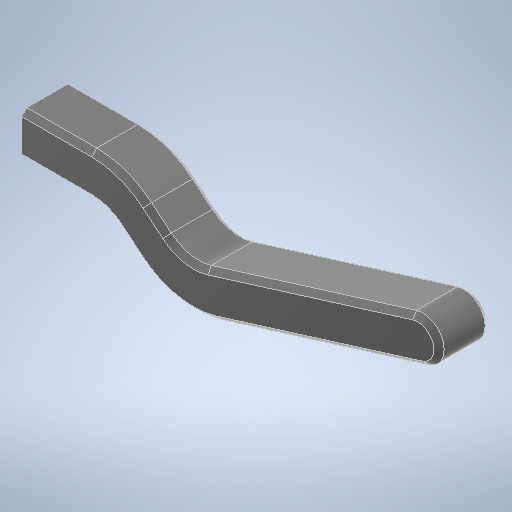
# Autodesk Inventor part: Robot_support
Saved by Autodesk Inventor 2025.2 (Build 292293000, 293)
## iProperties
Created: 2025-02-28
Part Number: Robot_support
Material: Generic
Document SubType Name: Modeling
Designer: Sergio Quintero
Density: 1 g/cm^3
Appearance: Smooth - Black
Author: Sergio Quintero
Autodesk Inventor part; units mm, degrees
ref_plane "YZ Plane" through (0, 0, 0) normal (1, 0, 0) x (0, 1, 0)
ref_plane "XZ Plane" through (0, 0, 0) normal (0, 1, 0) x (-1, 0, 0)
ref_plane "XY Plane" through (0, 0, 0) normal (0, 0, 1) x (1, 0, 0)
sketch "Sketch1" plane through (0, 0, 0) normal (0, 0, 1) x (1, 0, 0)
  line L0 (25, -12.5) -> (-25, -12.5)
  line L1 (-25, -12.5) -> (-25, 12.5)
  line L2 (-25, 12.5) -> (25, 12.5)
  line L3 (25, -12.5) -> (-25, 12.5) construction
  line L4 (-25, -12.5) -> (25, 12.5) construction
  line L5 (25, 12.5) -> (70, 12.5) construction
  line L6 (70, 12.5) -> (70, -17.5) construction
  line L7 (70, -17.5) -> (70, 27.5) construction
  line L8 (70, 27.5) -> (215, 27.5) construction
  line L9 (25, -12.5) -> (64.4199, -45.408)
  line L10 (70, -17.5) -> (41.0213, 6.6916)
  line L11 (70, -17.5) -> (215, 27.5)
  line L12 (215, 27.5) -> (222.41, 3.6234)
  line L13 (222.41, 3.6234) -> (77.41, -41.3766)
  line L14 (41.0213, 6.6916) -> (34.0635, 12.5)
  line L15 (25, 12.5) -> (34.0635, 12.5)
  line L16 (77.41, -41.3766) -> (64.4199, -45.408)
  point P0 (0, 0)
  dimension "d3" = 30
  dimension "d5" = 50
  dimension "d6" = 25
  dimension "d7" = 45
  dimension "d8" = 45
  dimension "d9" = 145
  dimension "d12" = 25
  dimension "d13" = 25
  constraints: 34 end point, 4 perpendicular, 3 parallel, 2 collinear, 2 horizontal, 2 midpoint, 1 point on line, 1 vertical
  measures "d3" distance of L6.end L5.end
  measures "d5" distance from line of L2.end L1
  measures "d6" distance between parallel lines of L0 L2
  measures "d7" distance from line of L6 L2.end
  measures "d8" distance of L6.end L7.end
  measures "d9" distance of L7.end L8.end
  measures "d12" distance of L8.end L12.end
  measures "d13" distance between parallel lines of L9 L10
extrude "Extrusion1" add sketch "Sketch1" along normal mid plane 30
fillet "Fillet1" radius 50 1 edges at (34.0635, 12.5, 0)
fillet "Fillet2" radius 25 1 edges at (25, -12.5, 0)
fillet "Fillet3" radius 50 1 edges at (64.4199, -45.408, 0)
fillet "Fillet4" radius 25 1 edges at (70, -17.5, 0)
fillet "Fillet5" radius 12.5 2 edges at (215, 27.5, 0) (222.41, 3.6234, 0)
chamfer "Chamfer1" distance 3 angle 45 26 edges at (32.9782, 9.5062, 15) (53.7689, -3.9502, 15) (70.6785, -14.1068, 15) (143.0259, 5.1632, 15) (212.5885, 22.9182, 15) (218.705, 15.5617, 15) (217.8282, 6.0349, 15) (150.4359, -18.7134, 15) (65.7768, -38.6215, 15) (37.7476, -23.1418, 15) (24.4573, -13.9969, 15) (-4.5318, -12.5, 15) (-4.5318, 12.5, 15) (32.9782, 9.5062, -15) (-4.5318, 12.5, -15) (53.7689, -3.9502, -15) (70.6785, -14.1068, -15) (143.0259, 5.1632, -15) (212.5885, 22.9182, -15) (218.705, 15.5617, -15) (217.8282, 6.0349, -15) (150.4359, -18.7134, -15) (65.7768, -38.6215, -15) (37.7476, -23.1418, -15) (24.4573, -13.9969, -15) (-4.5318, -12.5, -15)
body "Solid1"
